J4 (Autodesk Fusion 360 design; units mm, degrees)
part number: 2026-05-30-23-30-23-311
Autodesk Fusion 360 part; units mm, degrees
sketch "Sketch1" plane through (0, 0, 0) normal (0, 0, 1) x (1, 0, 0)
  line L0 (0, 0) -> (10, 0)
  line L1 (10, 0) -> (10, 10)
  line L2 (10, 10) -> (0, 10)
  line L3 (0, 10) -> (0, 0)
  dimension "d1" = 10
  dimension "d2" = 10
  constraint horizontal L0
  constraint vertical L1
  constraint horizontal L2
  constraint vertical L3
  constraint coincident L0.start L3.end
  measures "d1" distance of L0.start L0.end
  measures "d2" distance of L0.start L2.end
extrude "Extrude1" add sketch "Sketch1" along normal blind 25
sketch "Sketch2" plane through (0, 0, 0) normal (0, -1, 0) x (1, 0, 0)
  line L0 (0, 0) -> (10, 0)
  line L1 (10, 0) -> (10, 25)
  line L2 (10, 25) -> (0, 25)
  line L3 (0, 25) -> (0, 0)
  circle A0 centre (5, 20) radius 4
  dimension "d5" = 8
  measures "d5" diameter of A0
extrude "Extrude2" cut sketch "Sketch2" against normal blind 10 contours A0
sketch "Sketch3" plane through (0, 0, 0) normal (0, 0, -1) x (1, 0, 0)
  line L0 (0, 0) -> (0, -10)
  line L1 (0, -10) -> (10, -10)
  line L2 (10, -10) -> (10, 0)
  line L3 (10, 0) -> (0, 0)
  circle A0 centre (5, -5) radius 3.75
  dimension "d8" = 7.5
  measures "d8" diameter of A0
extrude "Extrude3" add sketch "Sketch3" along normal blind 10 contours A0
